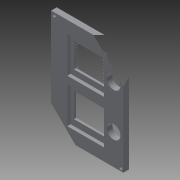
# Autodesk Inventor part: Face3
Saved by Autodesk Inventor 2015 (Build 190159000, 159)
## iProperties
Created: 2015-03-18
Part Number: Face3
Material: Generic
Document SubType Name: Modeling
Designer: ChristopherEvan
Density: 1 g/cm^3
Appearance: Default
Author: ChristopherEvan
Autodesk Inventor part; units mm, degrees
ref_plane "YZ Plane" through (0, 0, 0) normal (1, 0, 0) x (0, 1, 0)
ref_plane "XZ Plane" through (0, 0, 0) normal (0, 1, 0) x (-1, 0, 0)
ref_plane "XY Plane" through (0, 0, 0) normal (0, 0, 1) x (1, 0, 0)
sketch "Sketch1" plane through (0, 0, 0) normal (0, 0, 1) x (1, 0, 0)
  line L0 (62.5, 86.5) -> (62.5, 91.5) projected
  line L1 (62.5, 91.5) -> (57.5, 91.5) projected
  line L2 (62.5, -2.5) -> (62.5, 2.5) projected
  line L3 (57.5, -2.5) -> (62.5, -2.5) projected
  circle A0 centre (60, 0) radius 1.5 projected
  circle A1 centre (60, 89) radius 1.5 projected
  line L4 (-2.5, 91.5) -> (-2.5, 86.5) projected
  line L5 (2.5, 91.5) -> (-2.5, 91.5) projected
  circle A2 centre (0, 89) radius 1.5 projected
  line L6 (-2.5, 2.5) -> (-2.5, -2.5) projected
  line L7 (-2.5, -2.5) -> (2.5, -2.5) projected
  circle A3 centre (0, 0) radius 1.5 projected
  line L8 (62.5, 91.5) -> (-2.5, 91.5)
  line L9 (-2.5, 91.5) -> (-2.5, -2.5)
  line L10 (-2.5, -2.5) -> (62.5, -2.5)
  line L11 (62.5, -2.5) -> (62.5, 91.5)
  circle A4 centre (60, 89) radius 1.5
  circle A5 centre (60, 0) radius 1.5
  circle A6 centre (0, 0) radius 1.5
  circle A7 centre (0, 89) radius 1.5
  point P0 (0, 0)
  constraints: 8 end point, 4 centre point, 4 coincident, 4 concentric, 2 parallel, 1 horizontal, 1 perpendicular
sketch "Sketch1 outline for Extrusion1" plane through (0, 0, 0) normal (0, 0, 1) x (1, 0, 0)
  line L0 (62.5, -2.5) -> (62.5, 91.5)
  line L1 (-2.5, -2.5) -> (62.5, -2.5)
  line L2 (62.5, 91.5) -> (-2.5, 91.5)
  line L3 (-2.5, 91.5) -> (-2.5, -2.5)
  circle A0 centre (0, 0) radius 1.5
  circle A1 centre (60, 0) radius 1.5
  circle A2 centre (0, 89) radius 1.5
  circle A3 centre (60, 89) radius 1.5
extrude "Extrusion1" add sketch "Sketch1 outline for Extrusion1" along normal blind 5
sketch "Sketch2" plane through (0, 0, 5) normal (0, 0, 1) x (1, 0, 0)
  line L0 (45.035378, 80.435992) -> (12.035378, 80.435992)
  line L1 (45.035378, 47.935993) -> (45.035378, 80.435992)
  line L2 (12.035378, 47.935993) -> (45.035378, 47.935993)
  line L3 (12.035378, 80.435992) -> (12.035378, 47.935993)
  line L4 (45.035378, 80.435992) -> (12.035378, 80.435992)
  line L5 (12.035378, 80.435992) -> (12.035378, 47.935993)
  line L6 (12.035378, 47.935993) -> (45.035378, 47.935993)
  line L7 (45.035378, 47.935993) -> (45.035378, 80.435992)
  line L8 (62.5, 91.5) -> (-2.5, 91.5)
  line L9 (62.5, -2.5) -> (62.5, 91.5)
  line L10 (-2.5, 91.5) -> (-2.5, -2.5)
  line L11 (45.035378, 41.064007) -> (12.035378, 41.064007)
  line L12 (12.035378, 41.064007) -> (12.035378, 8.564008)
  line L13 (12.035378, 8.564008) -> (45.035378, 8.564008)
  line L14 (45.035378, 8.564008) -> (45.035378, 41.064007)
  line L15 (-2.5, -2.5) -> (62.5, -2.5)
  point P0 (0, 0)
  dimension "d2" = 11.06401
  dimension "d3" = 17.46462
  dimension "d4" = 14.53538
  dimension "d5" = 11.06401
  dimension "d6" = 17.46462
  dimension "d7" = 14.53538
  dimension "d8" = 32.5
  dimension "d9" = 32.5
  constraints: 24 end point, 2 parallel, 1 horizontal, 1 perpendicular
  measures "d2" distance between parallel lines of L8 L0
  measures "d3" distance between parallel lines of L9 L1
  measures "d4" distance between parallel lines of L10 L3
  measures "d5" distance between parallel lines of L15 L13
  measures "d6" distance between parallel lines of L9 L14
  measures "d7" distance between parallel lines of L10 L12
  measures "d8" distance between parallel lines of L6 L4
  measures "d9" distance between parallel lines of L13 L11
sketch "Sketch2 outline for Extrusion2" plane through (0, 0, 5) normal (0, 0, 1) x (1, 0, 0)
  line L0 (45.035378, 47.935993) -> (45.035378, 80.435992)
  line L1 (12.035378, 47.935993) -> (45.035378, 47.935993)
  line L2 (12.035378, 80.435992) -> (12.035378, 47.935993)
  line L3 (45.035378, 80.435992) -> (12.035378, 80.435992)
  line L4 (45.035378, 8.564008) -> (45.035378, 41.064007)
  line L5 (12.035378, 8.564008) -> (45.035378, 8.564008)
  line L6 (12.035378, 41.064007) -> (12.035378, 8.564008)
  line L7 (45.035378, 41.064007) -> (12.035378, 41.064007)
extrude "Extrusion2" cut sketch "Sketch2 outline for Extrusion2" against normal blind 3
sketch "Sketch3" plane through (0, 0, 2) normal (0, 0, 1) x (1, 0, 0)
  circle A0 centre (17.035378, 72.935993) radius 0.255
  circle A1 centre (17.035378, 72.935993) radius 0.255
  circle A2 centre (17.035378, 70.364564) radius 0.255
  circle A3 centre (17.035378, 67.793135) radius 0.255
  circle A4 centre (17.035378, 65.221707) radius 0.255
  circle A5 centre (17.035378, 62.650278) radius 0.255
  circle A6 centre (17.035378, 60.07885) radius 0.255
  circle A7 centre (17.035378, 57.507421) radius 0.255
  circle A8 centre (17.035378, 54.935993) radius 0.255
  circle A9 centre (41.035378, 54.935993) radius 0.255
  circle A10 centre (41.035378, 57.507421) radius 0.255
  circle A11 centre (41.035378, 60.07885) radius 0.255
  circle A12 centre (41.035378, 62.650278) radius 0.255
  circle A13 centre (41.035378, 65.221707) radius 0.255
  circle A14 centre (41.035378, 67.793135) radius 0.255
  circle A15 centre (41.035378, 70.364564) radius 0.255
  circle A16 centre (41.035378, 72.935993) radius 0.255
  line L0 (41.035378, 72.935993) -> (17.035378, 72.935993)
  line L1 (17.035378, 72.935993) -> (17.035378, 54.935993)
  line L2 (17.035378, 54.935993) -> (41.035378, 54.935993)
  line L3 (41.035378, 54.935993) -> (41.035378, 72.935993)
  line L4 (43.035378, 74.935993) -> (15.035378, 74.935993)
  line L5 (15.035378, 74.935993) -> (15.035378, 52.935993)
  line L6 (15.035378, 52.935993) -> (43.035378, 52.935993)
  line L7 (43.035378, 52.935993) -> (43.035378, 74.935993)
  line L8 (62.5, -2.5) -> (62.5, 91.5)
  line L9 (-2.5, 91.5) -> (-2.5, -2.5)
  line L10 (62.5, 44.5) -> (-2.5, 44.5)
  line L11 (62.5, 44.5) -> (-2.5, 44.5)
  line L12 (43.035378, 14.064007) -> (15.035378, 14.064007)
  line L13 (15.035378, 14.064007) -> (15.035378, 36.064007)
  line L14 (15.035378, 36.064007) -> (43.035378, 36.064007)
  line L15 (43.035378, 36.064007) -> (43.035378, 14.064007)
  point P0 (0, 0)
  dimension "d12" = 2
  dimension "d13" = 2
  dimension "d14" = 2
  dimension "d15" = 2
  constraints: 28 end point, 5 equal length, 4 symmetric about line, 2 horizontal, 2 midpoint, 2 perpendicular
  measures "d12" distance between parallel lines of L7 L3
  measures "d13" distance between parallel lines of L0 L4
  measures "d14" distance between parallel lines of L6 L2
  measures "d15" distance between parallel lines of L1 L5
sketch "Sketch3 outline for Extrusion3" plane through (0, 0, 2) normal (0, 0, 1) x (1, 0, 0)
  line L0 (43.035378, 52.935993) -> (43.035378, 74.935993)
  line L1 (43.035378, 74.935993) -> (15.035378, 74.935993)
  line L2 (15.035378, 74.935993) -> (15.035378, 52.935993)
  line L3 (15.035378, 52.935993) -> (43.035378, 52.935993)
  line L4 (41.035378, 54.935993) -> (40.780378, 54.935993)
  line L5 (41.035378, 55.190993) -> (41.035378, 54.935993)
  arc A0 (41.035378, 55.190993) -> (40.780378, 54.935993) centre (41.035378, 54.935993) cw
  line L6 (41.035378, 57.762421) -> (41.035378, 57.252421)
  arc A1 (41.035378, 57.762421) -> (41.035378, 57.252421) centre (41.035378, 57.507421) cw
  line L7 (41.035378, 60.33385) -> (41.035378, 59.82385)
  arc A2 (41.035378, 60.33385) -> (41.035378, 59.82385) centre (41.035378, 60.07885) cw
  line L8 (41.035378, 62.905278) -> (41.035378, 62.395278)
  arc A3 (41.035378, 62.905278) -> (41.035378, 62.395278) centre (41.035378, 62.650278) cw
  line L9 (41.035378, 65.476707) -> (41.035378, 64.966707)
  arc A4 (41.035378, 65.476707) -> (41.035378, 64.966707) centre (41.035378, 65.221707) cw
  line L10 (41.035378, 68.048135) -> (41.035378, 67.538135)
  arc A5 (41.035378, 68.048135) -> (41.035378, 67.538135) centre (41.035378, 67.793135) cw
  line L11 (41.035378, 70.619564) -> (41.035378, 70.109564)
  arc A6 (41.035378, 70.619564) -> (41.035378, 70.109564) centre (41.035378, 70.364564) cw
  line L12 (41.035378, 72.935993) -> (41.035378, 72.680993)
  line L13 (40.780378, 72.935993) -> (41.035378, 72.935993)
  arc A7 (40.780378, 72.935993) -> (41.035378, 72.680993) centre (41.035378, 72.935993) cw
  arc A8 (17.290378, 72.935993) -> (17.035378, 72.680993) centre (17.035378, 72.935993) ccw
  line L14 (17.035378, 72.935993) -> (17.290378, 72.935993)
  line L15 (17.035378, 72.680993) -> (17.035378, 72.935993)
  arc A9 (17.035378, 70.619564) -> (17.035378, 70.109564) centre (17.035378, 70.364564) ccw
  line L16 (17.035378, 70.109564) -> (17.035378, 70.619564)
  arc A10 (17.035378, 68.048135) -> (17.035378, 67.538135) centre (17.035378, 67.793135) ccw
  line L17 (17.035378, 67.538135) -> (17.035378, 68.048135)
  arc A11 (17.035378, 65.476707) -> (17.035378, 64.966707) centre (17.035378, 65.221707) ccw
  line L18 (17.035378, 64.966707) -> (17.035378, 65.476707)
  arc A12 (17.035378, 62.905278) -> (17.035378, 62.395278) centre (17.035378, 62.650278) ccw
  line L19 (17.035378, 62.395278) -> (17.035378, 62.905278)
  arc A13 (17.035378, 60.33385) -> (17.035378, 59.82385) centre (17.035378, 60.07885) ccw
  line L20 (17.035378, 59.82385) -> (17.035378, 60.33385)
  arc A14 (17.035378, 57.762421) -> (17.035378, 57.252421) centre (17.035378, 57.507421) ccw
  line L21 (17.035378, 57.252421) -> (17.035378, 57.762421)
  arc A15 (17.035378, 55.190993) -> (17.290378, 54.935993) centre (17.035378, 54.935993) ccw
  line L22 (17.035378, 54.935993) -> (17.035378, 55.190993)
  line L23 (17.290378, 54.935993) -> (17.035378, 54.935993)
  line L24 (43.035378, 14.064007) -> (43.035378, 36.064007)
  line L25 (15.035378, 14.064007) -> (43.035378, 14.064007)
  line L26 (15.035378, 36.064007) -> (15.035378, 14.064007)
  line L27 (43.035378, 36.064007) -> (15.035378, 36.064007)
extrude "Extrusion3" cut sketch "Sketch3 outline for Extrusion3" against normal up to next
sketch "Sketch4" plane through (0, 0, 5) normal (0, 0, 1) x (1, 0, 0)
  arc A0 (56.198928, 58.246466) -> (51.168338, 58.31708) centre (53.7624, 63.893219) ccw
  circle A1 centre (53.7624, 63.893219) radius 6.149999
  line L0 (45.035378, 47.935993) -> (45.035378, 79.935993)
  line L1 (62.5, -2.5) -> (62.5, 91.5)
  circle A2 centre (-10.97114, -10.97114) radius 6.149999
  line L2 (45.035378, 9.064007) -> (45.035378, 41.064007)
  point P0 (0, 0)
  dimension "d18" = 6.15
  dimension "d19" = 8.7376
  constraints: 3 centre point, 2 point on circle, 1 coincident
  measures "d18" radius of A0
  measures "d19" distance from line of L1 A0.centre
sketch "Sketch4 outline for Extrusion4" plane through (0, 0, 5) normal (0, 0, 1) x (1, 0, 0)
  circle A0 centre (53.7624, 63.893219) radius 6.149999
  circle A1 centre (-10.97114, -10.97114) radius 6.149999
extrude "Extrusion4" cut sketch "Sketch4 outline for Extrusion4" against normal up to next
sketch "Sketch5" plane through (0, 0, 5) normal (0, 0, 1) x (1, 0, 0)
  line L0 (62.5, -2.5) -> (62.5, 91.5)
  arc A0 (53.437399, 84.030969) -> (54.587399, 84.030969) centre (54.012399, 83.093219) ccw
  arc A1 (54.587399, 54.514655) -> (53.437399, 54.514655) centre (54.012399, 55.393219) ccw
  arc A2 (54.587399, 5.176256) -> (53.437399, 5.176256) centre (54.012399, 6.114006) ccw
  arc A3 (53.437399, 34.69257) -> (54.587399, 34.69257) centre (54.012399, 33.814006) ccw
  line L1 (59.712392, 80.493219) -> (48.312406, 80.493219)
  line L2 (48.312406, 8.714006) -> (59.712392, 8.714006)
  circle A4 centre (53.7624, 63.893219) radius 6.149999
  circle A5 centre (53.7624, 25.064007) radius 6.149999
  line L3 (59.912399, 57.74322) -> (47.612401, 57.74322)
  line L4 (47.612401, 57.74322) -> (47.612401, 80.493219)
  line L5 (47.612401, 80.493219) -> (59.912399, 80.493219)
  line L6 (59.912399, 80.493219) -> (59.912399, 57.74322)
  line L7 (59.912399, 31.214006) -> (47.612401, 31.214006)
  line L8 (47.612401, 31.214006) -> (47.612401, 8.464007)
  line L9 (47.612401, 8.464007) -> (59.912399, 8.464007)
  line L10 (59.912399, 8.464007) -> (59.912399, 31.214006)
  circle A6 centre (54.012399, 83.093219) radius 1.1
  circle A7 centre (54.012399, 55.393219) radius 1.05
  circle A8 centre (54.012399, 33.814006) radius 1.05
  circle A9 centre (54.012399, 6.114006) radius 1.1
  constraints: 16 end point, 4 centre point, 4 coincident, 4 concentric, 4 parallel, 2 horizontal, 2 perpendicular
sketch "Sketch5 outline for Extrusion5" plane through (0, 0, 5) normal (0, 0, 1) x (1, 0, 0)
  circle A0 centre (54.012399, 55.393219) radius 1.05
  circle A1 centre (54.012399, 33.814006) radius 1.05
  circle A2 centre (54.012399, 83.093219) radius 1.1
  circle A3 centre (54.012399, 6.114006) radius 1.1
  line L0 (59.912399, 57.74322) -> (47.612401, 57.74322)
  line L1 (47.612401, 57.74322) -> (47.612401, 80.493219)
  line L2 (47.612401, 80.493219) -> (59.912399, 80.493219)
  line L3 (59.912399, 80.493219) -> (59.912399, 57.74322)
  line L4 (59.912399, 8.464007) -> (59.912399, 31.214006)
  line L5 (47.612401, 8.464007) -> (59.912399, 8.464007)
  line L6 (47.612401, 31.214006) -> (47.612401, 8.464007)
  line L7 (59.912399, 31.214006) -> (47.612401, 31.214006)
extrude "Extrusion5" cut sketch "Sketch5 outline for Extrusion5" against normal up to next
equation "\"d5\" = d2"
equation "\"d9\" = d8"
body "Solid1"
